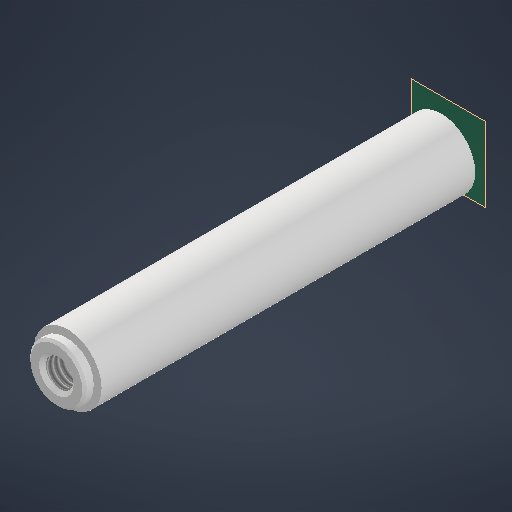
# Autodesk Inventor part: słupek
Saved by Autodesk Inventor 2026.1 (Build 301233020, 233B)
## iProperties
Created: 2026-03-16
Part Number: słupek
Material: Generic
Document SubType Name: Modeling
Designer: Jan
Density: 1 g/cm^3
Appearance: Default
Author: Jan
Autodesk Inventor part; units mm, degrees
ref_plane "YZ Plane" through (0, 0, 0) normal (1, 0, 0) x (0, 1, 0)
ref_plane "XZ Plane" through (0, 0, 0) normal (0, 1, 0) x (-1, 0, 0)
ref_plane "XY Plane" through (0, 0, 0) normal (0, 0, 1) x (1, 0, 0)
sketch "Sketch1" plane through (0, 0, 0) normal (0, 0, 1) x (1, 0, 0)
  circle A0 centre (0, 0) radius 3
  dimension "d0" = 6
  constraints: 1 centre point, 1 coincident
  measures "d0" diameter of A0
extrude "Extrusion1" add sketch "Sketch1" along normal blind 34.05
sketch "Sketch2" plane through (0, 0, 34.05) normal (0, 0, 1) x (1, 0, 0)
  circle A0 centre (0, 0) radius 2
  dimension "d3" = 4
  constraints: 1 centre point
  measures "d3" diameter of A0
hole "Hole1" at (0, 0, 34.05) direction (0, 0, -1) diameter 2.459 depth 8.8 tip angle 118 thread size "M3x0.5" class "6H" standard "ISO Metric profile"
chamfer "Chamfer1" distance 0.3 angle 45 1 edges at (0, 1.2295, 34.05)
sketch "Sketch3" plane through (0, 0, 34.05) normal (0, 0, 1) x (1, 0, 0)
  circle A0 centre (0, 0) radius 3
  circle A1 centre (0, 0) radius 2.5
  dimension "d14" = 5
  constraints: 2 centre point, 2 coincident
  measures "d14" diameter of A1
extrude "Extrusion2" cut sketch "Sketch3" against normal blind 1
sketch "Sketch4" plane through (0, 0, 0) normal (0, 0, -1) x (-1, 0, 0)
  circle A0 centre (0, 0) radius 1.5
  dimension "d17" = 3
  constraints: 1 centre point, 1 coincident
  measures "d17" diameter of A0
extrude "Extrusion3" add sketch "Sketch4" along normal blind 1
sketch "Sketch5" plane through (0, 0, -1) normal (0, 0, -1) x (-1, 0, 0)
  point P0 (0, 0)
  point P1 (0, 0)
  constraints: 1 coincident
hole "Hole2" at (0, 0, -1) direction (0, 0, 1) diameter 2 depth 2.5 tip angle 118
ref_plane "Work Plane2" through (0, 0, -0.5) normal (0, 0, -1) x (-1, 0, 0)
sketch "Sketch7" plane through (0, 0, -0.5) normal (0, 0, -1) x (-1, 0, 0)
  circle A0 centre (0, 0) radius 1.4
  circle A1 centre (0, 0) radius 1.5
  dimension "d29" = 2.8
  dimension "d30" = 3
  constraints: 2 centre point, 2 coincident
  measures "d29" diameter of A0
  measures "d30" diameter of A1
extrude "Extrusion4" cut sketch "Sketch7" against normal blind 0.5
sketch "Sketch8" plane through (0, 0, 33.05) normal (0, 0, 1) x (1, 0, 0)
  circle A0 centre (0, 0) radius 2.5
  circle A1 centre (0, 0) radius 2.5 projected
  circle A2 centre (0, 0) radius 2.3
  dimension "d31" = 4.6
  constraints: 2 centre point, 2 coincident
  measures "d31" diameter of A2
extrude "Extrusion5" cut sketch "Sketch8" along normal blind 0.2
chamfer "Chamfer2" distance 0.2 angle 45 2 edges at (1.5, 0, -1) (-2.5, 0, 34.05)
body "Solid1"
